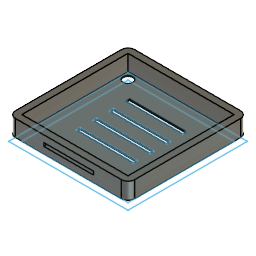
camplate (Autodesk Fusion 360 design; units mm, degrees)
part number: 2025-12-08-12-01-31-899
Autodesk Fusion 360 part; units mm, degrees
sketch "Sketch1" plane through (0, 0, 0) normal (0, 0, 1) x (1, 0, 0)
  line L0 (-27.6043, 30) -> (8.3957, 30)
  line L1 (8.3957, 30) -> (8.3957, -6)
  line L2 (8.3957, -6) -> (-27.6043, -6)
  line L3 (-27.6043, -6) -> (-27.6043, 30)
  line L4 (-25.6043, 28) -> (6.3957, 28)
  line L5 (6.3957, 28) -> (6.3957, -4)
  line L6 (6.3957, -4) -> (-25.6043, -4)
  line L7 (-25.6043, -4) -> (-25.6043, 28)
  dimension "d1" = 36
  dimension "d2" = 36
  dimension "d3" = 32
  dimension "d4" = 32
  dimension "d5" = 2
  dimension "d6" = 2
  constraint horizontal L0
  constraint vertical L1
  constraint horizontal L2
  constraint vertical L3
  constraint horizontal L4
  constraint vertical L5
  constraint horizontal L6
  constraint vertical L7
  measures "d1" distance of L0.start L2.end
  measures "d2" distance of L0.start L0.end
  measures "d3" distance of L4.start L6.end
  measures "d4" distance of L4.start L4.end
  measures "d5" distance of L0.start L4
  measures "d6" distance of L3 L4.start
extrude "Extrude1" add sketch "Sketch1" along normal blind 5 from surface at 2 makes body 1
sketch "Sketch2" plane through (0, 0, 2) normal (0, 0, -1) x (1, 0, 0)
  line L0 (-25.6043, 4) -> (6.3957, 4)
  line L1 (6.3957, 4) -> (6.3957, -28)
  line L2 (6.3957, -28) -> (-25.6043, -28)
  line L3 (-25.6043, -28) -> (-25.6043, 4)
  line L4 (8.3957, 6) -> (-27.6043, 6)
  line L5 (-27.6043, 6) -> (-27.6043, -30)
  line L6 (-27.6043, -30) -> (8.3957, -30)
  line L7 (8.3957, -30) -> (8.3957, 6)
extrude "Extrude2" add sketch "Sketch2" along normal blind 0.2 separate body contours L0 L1 L2 L3 makes body 2
move_body "Move1" bodies 2 to x (1, 0, 0) y (0, 1, 0) z (0, 0, 1) at (0, 0, 0.2)
fillet "Fillet1" radius 2 1 edges at (-27.6043, 30, 4.5) on bodies 1
fillet "Fillet2" radius 2 1 edges at (-27.6043, -6, 4.5) on bodies 1
fillet "Fillet3" radius 2 1 edges at (8.3957, -6, 4.5) on bodies 1
fillet "Fillet4" radius 2 1 edges at (8.3957, 30, 4.5) on bodies 1
extrude "Extrude3" add 1 faces at (-14.9376, 17.3333, 2) along direction (0, 0, -1) blind 0.1 on bodies 2 bodies 1 2
sketch "Sketch3" plane through (0, 0, 2.2) normal (0, 0, 1) x (-1, 0, 0)
  line L0 (-6.3957, -28) -> (25.6043, -28)
  line L1 (25.6043, -28) -> (25.6043, 4)
  line L2 (25.6043, 4) -> (-6.3957, 4)
  line L3 (-6.3957, 4) -> (-6.3957, -28)
  circle A0 centre (23.6043, 2) radius 1.5
  circle A1 centre (23.6043, 2) radius 2
  circle A2 centre (-4.3957, 2) radius 1.5
  circle A3 centre (-4.3957, 2) radius 2
  circle A4 centre (-4.3957, -26) radius 1.5
  circle A5 centre (-4.3957, -26) radius 2
  circle A6 centre (23.6043, -26) radius 1.5
  circle A7 centre (23.6043, -26) radius 2
  dimension "d22" = 3
  dimension "d23" = 4
  dimension "d24" = 3
  dimension "d25" = 4
  dimension "d26" = 3
  dimension "d27" = 4
  dimension "d28" = 3
  dimension "d29" = 4
  constraint coincident A0.centre A1.centre
  constraint tangent L1 A1
  constraint tangent L2 A1
  constraint coincident A6.centre A7.centre
  constraint tangent L0 A7
  constraint tangent L1 A7
  constraint coincident A4.centre A5.centre
  constraint tangent L0 A5
  constraint tangent L3 A5
  constraint coincident A2.centre A3.centre
  constraint tangent L3 A3
  constraint tangent L2 A3
  measures "d22" diameter of A0
  measures "d23" diameter of A1
  measures "d24" diameter of A2
  measures "d25" diameter of A3
  measures "d26" diameter of A4
  measures "d27" diameter of A5
  measures "d28" diameter of A6
  measures "d29" diameter of A7
extrude "Extrude4" cut sketch "Sketch3" against normal blind 0.4 contours A2 bodies 1
extrude "Extrude5" cut sketch "Sketch3" against normal blind 4 contours A0 bodies 1
extrude "Extrude6" cut sketch "Sketch3" against normal blind 4 contours A6 bodies 1
extrude "Extrude7" cut sketch "Sketch3" against normal blind 4 contours A4 bodies 1
sketch "Sketch4" plane through (0, -6, 0) normal (0, -1, 0) x (1, 0, 0)
  line L0 (6.3957, 2) -> (6.3957, 7)
  line L1 (6.3957, 7) -> (-25.6043, 7)
  line L2 (-25.6043, 7) -> (-25.6043, 2)
  line L3 (-25.6043, 2) -> (6.3957, 2)
  line L4 (-17, 5) -> (-2, 5)
  line L5 (-2, 5) -> (-2, 4)
  line L6 (-2, 4) -> (-17, 4)
  line L7 (-17, 4) -> (-17, 5)
  constraint horizontal L4
  constraint vertical L5
  constraint horizontal L6
  constraint vertical L7
extrude "Extrude8" cut sketch "Sketch4" against normal blind 5 contours L4 L5 L6 L7 bodies 1
sketch "Sketch5" plane through (0, 0, 2.2) normal (0, 0, 1) x (-1, 0, 0)
  circle A0 centre (-4.3957, -26) radius 1.5
  circle A1 centre (23.6043, -26) radius 1.5
  circle A2 centre (23.6043, 2) radius 1.5
  circle A3 centre (-4.3957, 2) radius 1.5
  line L0 (-6.3957, -28) -> (25.6043, -28)
  line L1 (25.6043, -28) -> (25.6043, 4)
  line L2 (25.6043, 4) -> (-6.3957, 4)
  line L3 (-6.3957, 4) -> (-6.3957, -28)
  line L4 (18, -16) -> (1, -16)
  line L5 (1, -16) -> (1, -15)
  line L6 (1, -15) -> (18, -15)
  line L7 (18, -15) -> (18, -16)
  line L8 (1, -11) -> (18, -11)
  line L9 (18, -11) -> (18, -10)
  line L10 (18, -10) -> (1, -10)
  line L11 (1, -10) -> (1, -11)
  line L12 (18, -6) -> (1, -6)
  line L13 (1, -6) -> (1, -5)
  line L14 (1, -5) -> (18, -5)
  line L15 (18, -5) -> (18, -6)
  line L16 (18.1043, -21) -> (1.1043, -21)
  line L17 (1.1043, -21) -> (1.1043, -20)
  line L18 (1.1043, -20) -> (18.1043, -20)
  line L19 (18.1043, -20) -> (18.1043, -21)
  dimension "d40" = 7
  dimension "d41" = 7.5
  dimension "d42" = 4
  dimension "d43" = 4
  dimension "d44" = 4
  constraint horizontal L4
  constraint vertical L5
  constraint horizontal L6
  constraint vertical L7
  constraint horizontal L8
  constraint vertical L9
  constraint horizontal L10
  constraint vertical L11
  constraint horizontal L12
  constraint vertical L13
  constraint horizontal L14
  constraint vertical L15
  constraint horizontal L16
  constraint vertical L17
  constraint horizontal L18
  constraint vertical L19
  measures "d40" distance of L0.end L16
  measures "d41" horizontal distance of L0.end L18.end
  measures "d42" distance of L4 L18.end
  measures "d43" distance of L6.end L8
  measures "d44" distance of L9.end L12
extrude "Extrude9" cut sketch "Sketch5" against normal blind 5 contours L16 L17 L18 L19 bodies 1
extrude "Extrude10" cut sketch "Sketch5" against normal blind 5 contours L4 L5 L6 L7 | L8 L9 L10 L11 | L12 L13 L14 L15 bodies 1
